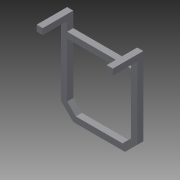
# Autodesk Inventor part: Base
Saved by Autodesk Inventor 2014 SP1 (Build 180222100, 222)
## iProperties
Created: 2013-12-26
Part Number: Base
Material: Generic
Document SubType Name: Modeling
Designer: tom
Density: 1 g/cm^3
Appearance: Default
Author: tom
Autodesk Inventor part; units mm, degrees
ref_plane "YZ Plane" through (0, 0, 0) normal (1, 0, 0) x (0, 1, 0)
ref_plane "XZ Plane" through (0, 0, 0) normal (0, 1, 0) x (-1, 0, 0)
ref_plane "XY Plane" through (0, 0, 0) normal (0, 0, 1) x (1, 0, 0)
sketch "Sketch1" plane through (0, 0, 0) normal (0, 0, 1) x (1, 0, 0)
  line L0 (0, 0) -> (146.05, 0) construction
  line L1 (146.05, 0) -> (146.05, 144.018) construction
  line L2 (146.05, 144.018) -> (0, 144.018) construction
  line L3 (0, 144.018) -> (0, 0) construction
  line L4 (-6.35, 150.368) -> (152.4, 150.368) construction
  line L5 (152.4, 182.118) -> (152.4, -6.35) construction
  line L6 (152.4, -6.35) -> (-6.35, -6.35) construction
  line L7 (-6.35, -6.35) -> (-6.35, 150.368) construction
  line L8 (6.35, 137.668) -> (139.7, 137.668) construction
  line L9 (139.7, 137.668) -> (139.7, 6.35) construction
  line L10 (139.7, 6.35) -> (6.35, 6.35) construction
  line L11 (6.35, 6.35) -> (6.35, 150.368) construction
  line L12 (152.4, 150.368) -> (139.7, 137.668) construction
  line L13 (-6.35, 150.368) -> (6.35, 137.668) construction
  line L14 (19.05, 124.968) -> (127, 124.968) construction
  line L15 (127, 124.968) -> (127, 19.05) construction
  line L16 (127, 19.05) -> (19.05, 19.05) construction
  line L17 (19.05, 19.05) -> (19.05, 124.968) construction
  line L18 (19.05, 150.368) -> (-6.35, 124.968) construction
  line L19 (24.3105, 137.668) -> (6.35, 119.7075) construction
  line L20 (73.025, 124.968) -> (73.025, 150.368) construction
  line L21 (19.05, 72.009) -> (-6.35, 72.009) construction
  line L22 (6.35, 150.368) -> (139.7, 150.368)
  line L23 (-6.35, 19.05) -> (19.05, -6.35)
  line L24 (19.05, -6.35) -> (127, -6.35)
  line L25 (6.35, 24.3105) -> (24.3105, 6.35)
  line L26 (24.3105, 6.35) -> (73.025, 6.35)
  line L27 (121.7395, 6.35) -> (73.025, 6.35)
  line L28 (152.4, 19.05) -> (127, -6.35)
  line L29 (139.7, 137.668) -> (139.7, 24.3105)
  line L30 (139.7, 24.3105) -> (121.7395, 6.35)
  line L31 (152.4, 182.118) -> (152.4, 19.05)
  line L32 (6.35, 137.668) -> (139.7, 137.668)
  line L33 (6.35, 137.668) -> (6.35, 24.3105)
  line L34 (-6.35, 19.05) -> (-6.35, 182.118)
  line L35 (6.35, 150.368) -> (6.35, 182.118)
  line L36 (6.35, 182.118) -> (-6.35, 182.118)
  line L37 (139.7, 150.368) -> (139.7, 182.118)
  line L38 (139.7, 182.118) -> (152.4, 182.118)
  point P0 (152.4, 124.968)
  point P1 (121.7395, 137.668)
  point P2 (139.7, 119.7075)
  point P3 (73.025, -6.35)
  point P4 (127, 150.368)
  dimension "d0" = 146.05
  dimension "d1" = 144.018
  dimension "d2" = 6.35
  dimension "d3" = 6.35
  dimension "d4" = 12.7
  dimension "d5" = 12.7
  constraints: 78 end point, 17 point on line, 16 symmetric about line, 12 perpendicular, 7 midpoint, 6 parallel, 1 collinear, 1 horizontal, 6 other
  measures "d0" distance of L0.start L0.end
  measures "d1" distance of L0.end L1.end
  measures "d2" distance between parallel lines of L2 L4
  measures "d3" distance between parallel lines of L8 L2
  measures "d4" distance between parallel lines of L8 L14
  measures "d5" distance between parallel lines of L18 L19
extrude "Extrusion1" add sketch "Sketch1" against normal blind 12.7
sketch "Sketch2" plane through (0, 0, 0) normal (0, 0, 1) x (1, 0, 0)
  line L0 (152.4, 182.118) -> (152.4, 19.05) projected
  line L1 (139.7, 182.118) -> (152.4, 182.118) projected
  line L2 (139.7, 150.368) -> (139.7, 182.118) projected
  line L3 (139.7, 169.418) -> (152.4, 169.418)
  line L4 (139.7, 169.418) -> (139.7, 182.118)
  line L5 (152.4, 182.118) -> (139.7, 182.118)
  line L6 (152.4, 182.118) -> (152.4, 180.5447)
  line L7 (152.4, 169.418) -> (152.4, 182.118)
  point P0 (0, 0)
  dimension "d10" = 12.7
  constraints: 10 end point, 2 collinear, 1 perpendicular, 1 point on line
  measures "d10" distance between parallel lines of L3 L1
extrude "Extrusion2" add sketch "Sketch2" along normal blind 50.8
sketch "Sketch3" plane through (0, 0, 0) normal (0, 0, 1) x (1, 0, 0)
  line L0 (6.35, 182.118) -> (6.35, 150.368) projected
  line L1 (-6.35, 182.118) -> (6.35, 182.118) projected
  line L2 (-6.35, 19.05) -> (-6.35, 182.118) projected
  line L3 (6.35, 169.418) -> (-6.35, 169.418)
  line L4 (-6.35, 169.418) -> (-6.35, 182.118)
  line L5 (6.35, 182.118) -> (6.35, 169.418)
  point P0 (0, 0)
  constraints: 6 end point, 2 collinear, 2 point on line
extrude "Extrusion3" add sketch "Sketch3" along normal up to surface (50.8 mm away)
body "Solid1"
